Autodesk Inventor part; units mm, degrees
(part 3 of 3)
ref_plane "to_Bolt_1_56_YZ" through (-142.1053, 0, -300) normal (1, 0, 0) x (0, 0, -1)
ref_plane "to_Bolt_1_56_ZX" through (-142.1053, 0, -300) normal (0, 0, -1) x (0, 1, 0)
ref_plane "to_Bolt_1_57_XY" through (-139.2344, 0, -300) normal (0, 1, 0) x (1, 0, 0)
ref_plane "to_Bolt_1_57_YZ" through (-139.2344, 0, -300) normal (1, 0, 0) x (0, 0, -1)
ref_plane "to_Bolt_1_57_ZX" through (-139.2344, 0, -300) normal (0, 0, -1) x (0, 1, 0)
ref_plane "to_Bolt_1_58_XY" through (-136.3636, 0, -300) normal (0, 1, 0) x (1, 0, 0)
ref_plane "to_Bolt_1_58_YZ" through (-136.3636, 0, -300) normal (1, 0, 0) x (0, 0, -1)
ref_plane "to_Bolt_1_58_ZX" through (-136.3636, 0, -300) normal (0, 0, -1) x (0, 1, 0)
ref_plane "to_Bolt_1_59_XY" through (-133.4928, 0, -300) normal (0, 1, 0) x (1, 0, 0)
ref_plane "to_Bolt_1_59_YZ" through (-133.4928, 0, -300) normal (1, 0, 0) x (0, 0, -1)
ref_plane "to_Bolt_1_59_ZX" through (-133.4928, 0, -300) normal (0, 0, -1) x (0, 1, 0)
ref_plane "to_Bolt_1_6_XY" through (-285.6459, 0, -300) normal (0, 1, 0) x (1, 0, 0)
ref_plane "to_Bolt_1_6_YZ" through (-285.6459, 0, -300) normal (1, 0, 0) x (0, 0, -1)
ref_plane "to_Bolt_1_6_ZX" through (-285.6459, 0, -300) normal (0, 0, -1) x (0, 1, 0)
ref_plane "to_Bolt_1_60_XY" through (-130.622, 0, -300) normal (0, 1, 0) x (1, 0, 0)
ref_plane "to_Bolt_1_60_YZ" through (-130.622, 0, -300) normal (1, 0, 0) x (0, 0, -1)
ref_plane "to_Bolt_1_60_ZX" through (-130.622, 0, -300) normal (0, 0, -1) x (0, 1, 0)
ref_plane "to_Bolt_1_61_XY" through (-127.7512, 0, -300) normal (0, 1, 0) x (1, 0, 0)
ref_plane "to_Bolt_1_61_YZ" through (-127.7512, 0, -300) normal (1, 0, 0) x (0, 0, -1)
ref_plane "to_Bolt_1_61_ZX" through (-127.7512, 0, -300) normal (0, 0, -1) x (0, 1, 0)
ref_plane "to_Bolt_1_62_XY" through (-124.8804, 0, -300) normal (0, 1, 0) x (1, 0, 0)
ref_plane "to_Bolt_1_62_YZ" through (-124.8804, 0, -300) normal (1, 0, 0) x (0, 0, -1)
ref_plane "to_Bolt_1_62_ZX" through (-124.8804, 0, -300) normal (0, 0, -1) x (0, 1, 0)
ref_plane "to_Bolt_1_63_XY" through (-122.0096, 0, -300) normal (0, 1, 0) x (1, 0, 0)
ref_plane "to_Bolt_1_63_YZ" through (-122.0096, 0, -300) normal (1, 0, 0) x (0, 0, -1)
ref_plane "to_Bolt_1_63_ZX" through (-122.0096, 0, -300) normal (0, 0, -1) x (0, 1, 0)
ref_plane "to_Bolt_1_64_XY" through (-119.1388, 0, -300) normal (0, 1, 0) x (1, 0, 0)
ref_plane "to_Bolt_1_64_YZ" through (-119.1388, 0, -300) normal (1, 0, 0) x (0, 0, -1)
ref_plane "to_Bolt_1_64_ZX" through (-119.1388, 0, -300) normal (0, 0, -1) x (0, 1, 0)
ref_plane "to_Bolt_1_65_XY" through (-116.2679, 0, -300) normal (0, 1, 0) x (1, 0, 0)
ref_plane "to_Bolt_1_65_YZ" through (-116.2679, 0, -300) normal (1, 0, 0) x (0, 0, -1)
ref_plane "to_Bolt_1_65_ZX" through (-116.2679, 0, -300) normal (0, 0, -1) x (0, 1, 0)
ref_plane "to_Bolt_1_66_XY" through (-113.3971, 0, -300) normal (0, 1, 0) x (1, 0, 0)
ref_plane "to_Bolt_1_66_YZ" through (-113.3971, 0, -300) normal (1, 0, 0) x (0, 0, -1)
ref_plane "to_Bolt_1_66_ZX" through (-113.3971, 0, -300) normal (0, 0, -1) x (0, 1, 0)
ref_plane "to_Bolt_1_67_XY" through (-110.5263, 0, -300) normal (0, 1, 0) x (1, 0, 0)
ref_plane "to_Bolt_1_67_YZ" through (-110.5263, 0, -300) normal (1, 0, 0) x (0, 0, -1)
ref_plane "to_Bolt_1_67_ZX" through (-110.5263, 0, -300) normal (0, 0, -1) x (0, 1, 0)
ref_plane "to_Bolt_1_68_XY" through (-107.6555, 0, -300) normal (0, 1, 0) x (1, 0, 0)
ref_plane "to_Bolt_1_68_YZ" through (-107.6555, 0, -300) normal (1, 0, 0) x (0, 0, -1)
ref_plane "to_Bolt_1_68_ZX" through (-107.6555, 0, -300) normal (0, 0, -1) x (0, 1, 0)
ref_plane "to_Bolt_1_69_XY" through (-104.7847, 0, -300) normal (0, 1, 0) x (1, 0, 0)
ref_plane "to_Bolt_1_69_YZ" through (-104.7847, 0, -300) normal (1, 0, 0) x (0, 0, -1)
ref_plane "to_Bolt_1_69_ZX" through (-104.7847, 0, -300) normal (0, 0, -1) x (0, 1, 0)
ref_plane "to_Bolt_1_7_XY" through (-282.7751, 0, -300) normal (0, 1, 0) x (1, 0, 0)
ref_plane "to_Bolt_1_7_YZ" through (-282.7751, 0, -300) normal (1, 0, 0) x (0, 0, -1)
ref_plane "to_Bolt_1_7_ZX" through (-282.7751, 0, -300) normal (0, 0, -1) x (0, 1, 0)
ref_plane "to_Bolt_1_70_XY" through (-101.9139, 0, -300) normal (0, 1, 0) x (1, 0, 0)
ref_plane "to_Bolt_1_70_YZ" through (-101.9139, 0, -300) normal (1, 0, 0) x (0, 0, -1)
ref_plane "to_Bolt_1_70_ZX" through (-101.9139, 0, -300) normal (0, 0, -1) x (0, 1, 0)
ref_plane "to_Bolt_1_71_XY" through (-99.0431, 0, -300) normal (0, 1, 0) x (1, 0, 0)
ref_plane "to_Bolt_1_71_YZ" through (-99.0431, 0, -300) normal (1, 0, 0) x (0, 0, -1)
ref_plane "to_Bolt_1_71_ZX" through (-99.0431, 0, -300) normal (0, 0, -1) x (0, 1, 0)
ref_plane "to_Bolt_1_72_XY" through (-96.1722, 0, -300) normal (0, 1, 0) x (1, 0, 0)
ref_plane "to_Bolt_1_72_YZ" through (-96.1722, 0, -300) normal (1, 0, 0) x (0, 0, -1)
ref_plane "to_Bolt_1_72_ZX" through (-96.1722, 0, -300) normal (0, 0, -1) x (0, 1, 0)
ref_plane "to_Bolt_1_73_XY" through (-93.3014, 0, -300) normal (0, 1, 0) x (1, 0, 0)
ref_plane "to_Bolt_1_73_YZ" through (-93.3014, 0, -300) normal (1, 0, 0) x (0, 0, -1)
ref_plane "to_Bolt_1_73_ZX" through (-93.3014, 0, -300) normal (0, 0, -1) x (0, 1, 0)
ref_plane "to_Bolt_1_74_XY" through (-90.4306, 0, -300) normal (0, 1, 0) x (1, 0, 0)
ref_plane "to_Bolt_1_74_YZ" through (-90.4306, 0, -300) normal (1, 0, 0) x (0, 0, -1)
ref_plane "to_Bolt_1_74_ZX" through (-90.4306, 0, -300) normal (0, 0, -1) x (0, 1, 0)
ref_plane "to_Bolt_1_75_XY" through (-87.5598, 0, -300) normal (0, 1, 0) x (1, 0, 0)
ref_plane "to_Bolt_1_75_YZ" through (-87.5598, 0, -300) normal (1, 0, 0) x (0, 0, -1)
ref_plane "to_Bolt_1_75_ZX" through (-87.5598, 0, -300) normal (0, 0, -1) x (0, 1, 0)
ref_plane "to_Bolt_1_76_XY" through (-84.689, 0, -300) normal (0, 1, 0) x (1, 0, 0)
ref_plane "to_Bolt_1_76_YZ" through (-84.689, 0, -300) normal (1, 0, 0) x (0, 0, -1)
ref_plane "to_Bolt_1_76_ZX" through (-84.689, 0, -300) normal (0, 0, -1) x (0, 1, 0)
ref_plane "to_Bolt_1_77_XY" through (-81.8182, 0, -300) normal (0, 1, 0) x (1, 0, 0)
ref_plane "to_Bolt_1_77_YZ" through (-81.8182, 0, -300) normal (1, 0, 0) x (0, 0, -1)
ref_plane "to_Bolt_1_77_ZX" through (-81.8182, 0, -300) normal (0, 0, -1) x (0, 1, 0)
ref_plane "to_Bolt_1_78_XY" through (-78.9474, 0, -300) normal (0, 1, 0) x (1, 0, 0)
ref_plane "to_Bolt_1_78_YZ" through (-78.9474, 0, -300) normal (1, 0, 0) x (0, 0, -1)
ref_plane "to_Bolt_1_78_ZX" through (-78.9474, 0, -300) normal (0, 0, -1) x (0, 1, 0)
ref_plane "to_Bolt_1_79_XY" through (-76.0766, 0, -300) normal (0, 1, 0) x (1, 0, 0)
ref_plane "to_Bolt_1_79_YZ" through (-76.0766, 0, -300) normal (1, 0, 0) x (0, 0, -1)
ref_plane "to_Bolt_1_79_ZX" through (-76.0766, 0, -300) normal (0, 0, -1) x (0, 1, 0)
ref_plane "to_Bolt_1_8_XY" through (-279.9043, 0, -300) normal (0, 1, 0) x (1, 0, 0)
ref_plane "to_Bolt_1_8_YZ" through (-279.9043, 0, -300) normal (1, 0, 0) x (0, 0, -1)
ref_plane "to_Bolt_1_8_ZX" through (-279.9043, 0, -300) normal (0, 0, -1) x (0, 1, 0)
ref_plane "to_Bolt_1_80_XY" through (-73.2057, 0, -300) normal (0, 1, 0) x (1, 0, 0)
ref_plane "to_Bolt_1_80_YZ" through (-73.2057, 0, -300) normal (1, 0, 0) x (0, 0, -1)
ref_plane "to_Bolt_1_80_ZX" through (-73.2057, 0, -300) normal (0, 0, -1) x (0, 1, 0)
ref_plane "to_Bolt_1_81_XY" through (-70.3349, 0, -300) normal (0, 1, 0) x (1, 0, 0)
ref_plane "to_Bolt_1_81_YZ" through (-70.3349, 0, -300) normal (1, 0, 0) x (0, 0, -1)
ref_plane "to_Bolt_1_81_ZX" through (-70.3349, 0, -300) normal (0, 0, -1) x (0, 1, 0)
ref_plane "to_Bolt_1_82_XY" through (-67.4641, 0, -300) normal (0, 1, 0) x (1, 0, 0)
ref_plane "to_Bolt_1_82_YZ" through (-67.4641, 0, -300) normal (1, 0, 0) x (0, 0, -1)
ref_plane "to_Bolt_1_82_ZX" through (-67.4641, 0, -300) normal (0, 0, -1) x (0, 1, 0)
ref_plane "to_Bolt_1_83_XY" through (-64.5933, 0, -300) normal (0, 1, 0) x (1, 0, 0)
ref_plane "to_Bolt_1_83_YZ" through (-64.5933, 0, -300) normal (1, 0, 0) x (0, 0, -1)
ref_plane "to_Bolt_1_83_ZX" through (-64.5933, 0, -300) normal (0, 0, -1) x (0, 1, 0)
ref_plane "to_Bolt_1_84_XY" through (-61.7225, 0, -300) normal (0, 1, 0) x (1, 0, 0)
ref_plane "to_Bolt_1_84_YZ" through (-61.7225, 0, -300) normal (1, 0, 0) x (0, 0, -1)
ref_plane "to_Bolt_1_84_ZX" through (-61.7225, 0, -300) normal (0, 0, -1) x (0, 1, 0)
ref_plane "to_Bolt_1_85_XY" through (-58.8517, 0, -300) normal (0, 1, 0) x (1, 0, 0)
ref_plane "to_Bolt_1_85_YZ" through (-58.8517, 0, -300) normal (1, 0, 0) x (0, 0, -1)
ref_plane "to_Bolt_1_85_ZX" through (-58.8517, 0, -300) normal (0, 0, -1) x (0, 1, 0)
ref_plane "to_Bolt_1_86_XY" through (-55.9809, 0, -300) normal (0, 1, 0) x (1, 0, 0)
ref_plane "to_Bolt_1_86_YZ" through (-55.9809, 0, -300) normal (1, 0, 0) x (0, 0, -1)
ref_plane "to_Bolt_1_86_ZX" through (-55.9809, 0, -300) normal (0, 0, -1) x (0, 1, 0)
ref_plane "to_Bolt_1_87_XY" through (-53.11, 0, -300) normal (0, 1, 0) x (1, 0, 0)
ref_plane "to_Bolt_1_87_YZ" through (-53.11, 0, -300) normal (1, 0, 0) x (0, 0, -1)
ref_plane "to_Bolt_1_87_ZX" through (-53.11, 0, -300) normal (0, 0, -1) x (0, 1, 0)
ref_plane "to_Bolt_1_88_XY" through (-50.2392, 0, -300) normal (0, 1, 0) x (1, 0, 0)
ref_plane "to_Bolt_1_88_YZ" through (-50.2392, 0, -300) normal (1, 0, 0) x (0, 0, -1)
ref_plane "to_Bolt_1_88_ZX" through (-50.2392, 0, -300) normal (0, 0, -1) x (0, 1, 0)
ref_plane "to_Bolt_1_89_XY" through (-47.3684, 0, -300) normal (0, 1, 0) x (1, 0, 0)
ref_plane "to_Bolt_1_89_YZ" through (-47.3684, 0, -300) normal (1, 0, 0) x (0, 0, -1)
ref_plane "to_Bolt_1_89_ZX" through (-47.3684, 0, -300) normal (0, 0, -1) x (0, 1, 0)
ref_plane "to_Bolt_1_9_XY" through (-277.0335, 0, -300) normal (0, 1, 0) x (1, 0, 0)
ref_plane "to_Bolt_1_9_YZ" through (-277.0335, 0, -300) normal (1, 0, 0) x (0, 0, -1)
ref_plane "to_Bolt_1_9_ZX" through (-277.0335, 0, -300) normal (0, 0, -1) x (0, 1, 0)
ref_plane "to_Bolt_1_90_XY" through (-44.4976, 0, -300) normal (0, 1, 0) x (1, 0, 0)
ref_plane "to_Bolt_1_90_YZ" through (-44.4976, 0, -300) normal (1, 0, 0) x (0, 0, -1)
ref_plane "to_Bolt_1_90_ZX" through (-44.4976, 0, -300) normal (0, 0, -1) x (0, 1, 0)
ref_plane "to_Bolt_1_91_XY" through (-41.6268, 0, -300) normal (0, 1, 0) x (1, 0, 0)
ref_plane "to_Bolt_1_91_YZ" through (-41.6268, 0, -300) normal (1, 0, 0) x (0, 0, -1)
ref_plane "to_Bolt_1_91_ZX" through (-41.6268, 0, -300) normal (0, 0, -1) x (0, 1, 0)
ref_plane "to_Bolt_1_92_XY" through (-38.756, 0, -300) normal (0, 1, 0) x (1, 0, 0)
ref_plane "to_Bolt_1_92_YZ" through (-38.756, 0, -300) normal (1, 0, 0) x (0, 0, -1)
ref_plane "to_Bolt_1_92_ZX" through (-38.756, 0, -300) normal (0, 0, -1) x (0, 1, 0)
ref_plane "to_Bolt_1_93_XY" through (-35.8852, 0, -300) normal (0, 1, 0) x (1, 0, 0)
ref_plane "to_Bolt_1_93_YZ" through (-35.8852, 0, -300) normal (1, 0, 0) x (0, 0, -1)
ref_plane "to_Bolt_1_93_ZX" through (-35.8852, 0, -300) normal (0, 0, -1) x (0, 1, 0)
ref_plane "to_Bolt_1_94_XY" through (-33.0144, 0, -300) normal (0, 1, 0) x (1, 0, 0)
ref_plane "to_Bolt_1_94_YZ" through (-33.0144, 0, -300) normal (1, 0, 0) x (0, 0, -1)
ref_plane "to_Bolt_1_94_ZX" through (-33.0144, 0, -300) normal (0, 0, -1) x (0, 1, 0)
ref_plane "to_Bolt_1_95_XY" through (-30.1435, 0, -300) normal (0, 1, 0) x (1, 0, 0)
ref_plane "to_Bolt_1_95_YZ" through (-30.1435, 0, -300) normal (1, 0, 0) x (0, 0, -1)
ref_plane "to_Bolt_1_95_ZX" through (-30.1435, 0, -300) normal (0, 0, -1) x (0, 1, 0)
ref_plane "to_Bolt_1_96_XY" through (-27.2727, 0, -300) normal (0, 1, 0) x (1, 0, 0)
ref_plane "to_Bolt_1_96_YZ" through (-27.2727, 0, -300) normal (1, 0, 0) x (0, 0, -1)
ref_plane "to_Bolt_1_96_ZX" through (-27.2727, 0, -300) normal (0, 0, -1) x (0, 1, 0)
ref_plane "to_Bolt_1_97_XY" through (-24.4019, 0, -300) normal (0, 1, 0) x (1, 0, 0)
ref_plane "to_Bolt_1_97_YZ" through (-24.4019, 0, -300) normal (1, 0, 0) x (0, 0, -1)
ref_plane "to_Bolt_1_97_ZX" through (-24.4019, 0, -300) normal (0, 0, -1) x (0, 1, 0)
ref_plane "to_Bolt_1_98_XY" through (-21.5311, 0, -300) normal (0, 1, 0) x (1, 0, 0)
ref_plane "to_Bolt_1_98_YZ" through (-21.5311, 0, -300) normal (1, 0, 0) x (0, 0, -1)
ref_plane "to_Bolt_1_98_ZX" through (-21.5311, 0, -300) normal (0, 0, -1) x (0, 1, 0)
ref_plane "to_Bolt_1_99_XY" through (-18.6603, 0, -300) normal (0, 1, 0) x (1, 0, 0)
ref_plane "to_Bolt_1_99_YZ" through (-18.6603, 0, -300) normal (1, 0, 0) x (0, 0, -1)
ref_plane "to_Bolt_1_99_ZX" through (-18.6603, 0, -300) normal (0, 0, -1) x (0, 1, 0)
ref_plane "to_Bolt_2_XY" through (300, 0, -300) normal (0, 1, 0) x (1, 0, 0)
ref_plane "to_Bolt_2_YZ" through (300, 0, -300) normal (1, 0, 0) x (0, 0, -1)
ref_plane "to_Bolt_2_ZX" through (300, 0, -300) normal (0, 0, -1) x (0, 1, 0)
ref_plane "to_Bolt_3_XY" through (-300, 0, 300) normal (0, 1, 0) x (1, 0, 0)
ref_plane "to_Bolt_3_YZ" through (-300, 0, 300) normal (1, 0, 0) x (0, 0, -1)
ref_plane "to_Bolt_3_ZX" through (-300, 0, 300) normal (0, 0, -1) x (0, 1, 0)
ref_plane "to_Bolt_4_XY" through (300, 0, 300) normal (0, 1, 0) x (1, 0, 0)
ref_plane "to_Bolt_4_YZ" through (300, 0, 300) normal (1, 0, 0) x (0, 0, -1)
ref_plane "to_Bolt_4_ZX" through (300, 0, 300) normal (0, 0, -1) x (0, 1, 0)
body "Solid1"
